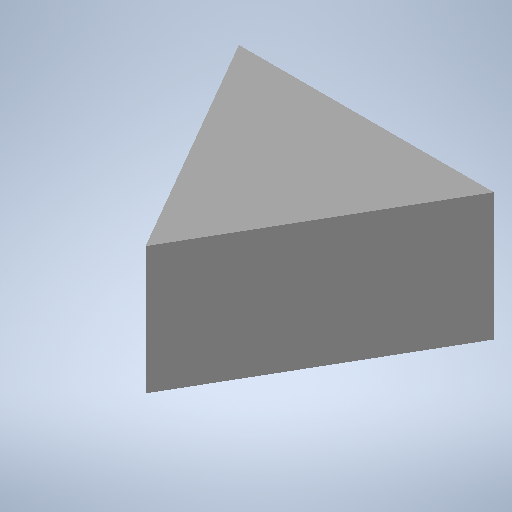
# Autodesk Inventor part: RT_FRM_008_PR_CenterTriangle
Saved by Autodesk Inventor 2025.4 (Build 294407000, 407)
## iProperties
Created: 2026-05-15
Part Number: RT_FRM_008_PR_CenterTriangle
Material: Générique
Document SubType Name: Modeling
Designer: louis
Density: 1 g/cm^3
Appearance: Par défaut
Author: louis
Autodesk Inventor part; units mm, degrees
ref_plane "YZ Plane" through (0, 0, 0) normal (1, 0, 0) x (0, 1, 0)
ref_plane "XZ Plane" through (0, 0, 0) normal (0, 1, 0) x (-1, 0, 0)
ref_plane "XY Plane" through (0, 0, 0) normal (0, 0, 1) x (1, 0, 0)
sketch "Sketch2" plane through (0, 0, 0) normal (0, 0, 1) x (1, 0, 0)
  line L0 (-40, 23.094) -> (40, 23.094)
  line L1 (40, 23.094) -> (0, -46.188)
  line L2 (0, -46.188) -> (-40, 23.094)
  line L3 (0, 23.094) -> (0, 0) construction
  line L4 (0, 0) -> (-20, -11.547) construction
  line L5 (0, 0) -> (20, -11.547) construction
  line L6 (26.1436, 18.094) -> (-26.1436, 18.094)
  line L7 (-28.7417, 13.594) -> (-2.5981, -31.688)
  line L8 (2.5981, -31.688) -> (28.7417, 13.594)
  arc A0 (-26.1436, 18.094) -> (-28.7417, 13.594) centre (-26.1436, 15.094) ccw
  arc A1 (28.7417, 13.594) -> (26.1436, 18.094) centre (26.1436, 15.094) ccw
  arc A2 (-2.5981, -31.688) -> (2.5981, -31.688) centre (0, -30.188) ccw
  dimension "d0" = 80
  dimension "d1" = 5
  dimension "d2" = 3
  constraints: 18 end point, 6 point on circle, 6 tangent, 4 equal length, 3 centre point, 3 midpoint, 2 equal radius, 1 horizontal, 2 other
  measures "d0" distance of L0.start L0.end
  measures "d1" distance between parallel lines of L0 L6
  measures "d2" radius of A0
extrude "Extrusion1" add sketch "Sketch2" along normal blind 10 contours L0 L1 L2 | A1 L8 A2 L7 A0 L6
extrude "Extrusion2" add sketch "Sketch2" against normal blind 30
body "Solid1"
